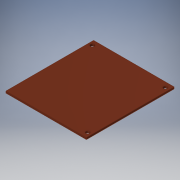
# Autodesk Inventor part: PCB
Saved by Autodesk Inventor 2019 (Build 230136000, 136)
## iProperties
Created: 2019-03-10
Part Number: PCB
Material: Copper
Document SubType Name: Modeling
Designer: savo
Density: 8.94 g/cm^3
Appearance: Copper - Satin
Author: savo
Autodesk Inventor part; units mm, degrees
ref_plane "YZ Plane" through (0, 0, 0) normal (1, 0, 0) x (0, 1, 0)
sketch "Sketch1" plane through (0, 0, 0) normal (0, 1, 0) x (-1, 0, 0)
  line L0 (0, 0) -> (-71.12, 0)
  line L1 (-71.12, 0) -> (-71.12, -77.47)
  line L2 (-71.12, -77.47) -> (0, -77.47)
  line L3 (0, -77.47) -> (0, 0)
  dimension "d0" = 71.12
  dimension "d1" = 77.47
  constraints: 8 end point, 2 parallel, 1 horizontal, 1 perpendicular
  measures "d0" distance of L2.end L1.end
  measures "d1" distance of L1.end L0.end
extrude "Extrusion1" add sketch "Sketch1" along normal blind 1.6
sketch "Sketch2" plane through (0, 1.6, 0) normal (0, 1, 0) x (1, 0, 0)
  line L0 (67.818, 4.445) -> (3.302, 4.445) construction
  line L1 (3.302, 4.445) -> (3.302, 73.025) construction
  line L2 (3.302, 73.025) -> (67.818, 73.025) construction
  line L3 (67.818, 73.025) -> (67.818, 4.445) construction
  line L4 (0, 0) -> (71.12, 0) construction
  line L5 (35.56, 0) -> (35.56, 77.47) construction
  line L6 (71.12, 77.47) -> (0, 77.47) construction
  line L7 (67.818, 73.025) -> (3.302, 4.445) construction
  point P0 (35.56, 38.735)
  dimension "d4" = 68.58
  dimension "d5" = 64.516
  constraints: 12 end point, 4 midpoint, 3 coincident, 2 parallel, 1 horizontal, 1 perpendicular
  measures "d4" distance of L2.end L0.start
  measures "d5" distance of L1.end L2.end
hole "Hole1" at (3.302, 1.6, -73.025) at (67.818, 1.6, -4.445) at (67.818, 1.6, -73.025) direction (0, -1, 0) diameter 3.4 end through all clearance for "Flat Head Machine Screw" size "M3" standard "Ansi Metric M Profile"
ref_plane "Work Plane1" through (0, 0, -38.735) normal (0, 0, 1) x (1, 0, 0)
ref_plane "Work Plane2" through (35.56, 0, -77.47) normal (-1, 0, 0) x (0, 0, 1)
body "Solid1"
